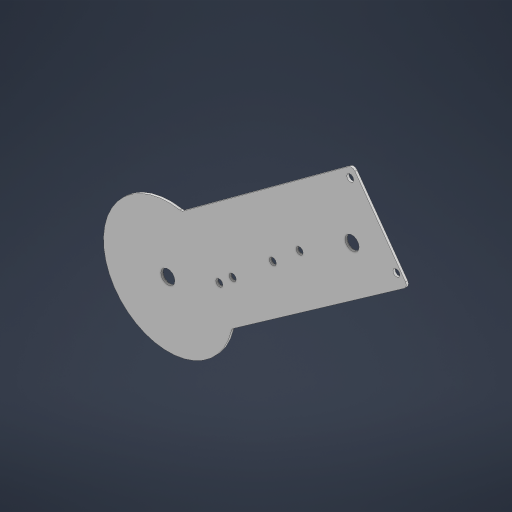
# Autodesk Inventor part: Intake poly
Saved by Autodesk Inventor 2023.4 (Build 274418000, 418)
## iProperties
Created: 2023-12-15
Part Number: Intake poly
Material: Generic
Document SubType Name: Modeling
Designer: diego
Density: 1 g/cm^3
Appearance: Default
Author: diego
Autodesk Inventor part; units mm, degrees
ref_plane "YZ Plane" through (0, 0, 0) normal (1, 0, 0) x (0, 1, 0)
ref_plane "XZ Plane" through (0, 0, 0) normal (0, 1, 0) x (-1, 0, 0)
ref_plane "XY Plane" through (0, 0, 0) normal (0, 0, 1) x (1, 0, 0)
sketch "Sketch2" plane through (0, 0, 0) normal (0, 0, 1) x (1, 0, 0)
  circle A0 centre (-65.2715, -43.4254) radius 46.99
  line L0 (-19.2425, -52.8797) -> (108.4608, 36.9121)
  line L1 (108.4608, 36.9121) -> (68.0869, 93.186)
  line L2 (68.0869, 93.186) -> (-55.5981, 2.5581)
  circle A1 centre (100.0461, 41.8214) radius 2.54
  circle A2 centre (66.5651, 84.6941) radius 2.54
  circle A3 centre (-65.5862, -43.4643) radius 5.08
  circle A4 centre (67.9257, 44.5075) radius 5.08
  circle A5 centre (29.8863, 20.6511) radius 2.54
  circle A6 centre (10.4927, 4.2484) radius 2.54
  circle A7 centre (-18.5977, -20.3557) radius 2.54
  circle A8 centre (-28.2944, -28.557) radius 2.54
  point P0 (0, 0)
  dimension "d45" = 93.98
  dimension "d46" = 127.7033
  dimension "d47" = 153.3343
  dimension "d48" = 5.08
  dimension "d49" = 5.08
  dimension "d50" = 10.16
  dimension "d51" = 10.16
  dimension "d52" = 5.08
  dimension "d53" = 5.08
  dimension "d54" = 5.08
  dimension "d55" = 5.08
  constraints: 9 centre point, 6 end point, 2 point on circle
  measures "d45" diameter of A0
  measures "d46" horizontal distance of L0.start L0.end
  measures "d47" distance of L1.end L2.end
  measures "d48" diameter of A1
  measures "d49" diameter of A2
  measures "d50" diameter of A3
  measures "d51" diameter of A4
  measures "d52" diameter of A5
  measures "d53" diameter of A6
  measures "d54" diameter of A7
  measures "d55" diameter of A8
extrude "Extrusion2" add sketch "Sketch2" along normal blind 1.5875
fillet "Fillet2" radius 3.175 4 edges at (-55.5981, 2.5581, 0.7937) (68.0869, 93.186, 0.7937) (108.4608, 36.9121, 0.7937) (-19.2425, -52.8797, 0.7937)
body "Solid2"
